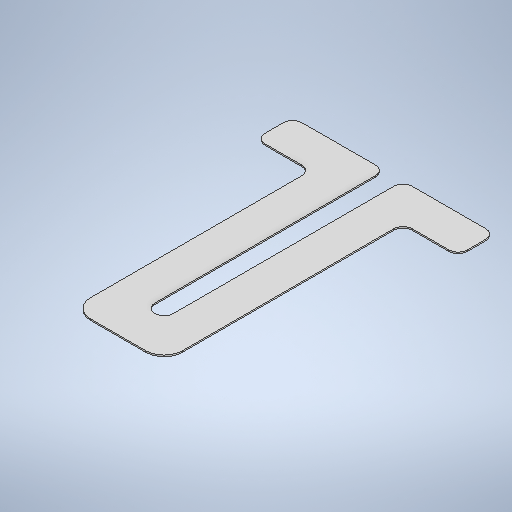
# Autodesk Inventor part: Part1
Saved by Autodesk Inventor 2025.4 (Build 294407000, 407)
## iProperties
Created: 2026-04-15
Part Number: Part1
Material: Generic
Document SubType Name: Modeling
Designer: gdira
Density: 1 g/cm^3
Appearance: Default
Author: gdira
Autodesk Inventor part; units mm, degrees
ref_plane "YZ Plane" through (0, 0, 0) normal (1, 0, 0) x (0, 1, 0)
ref_plane "XZ Plane" through (0, 0, 0) normal (0, 1, 0) x (-1, 0, 0)
ref_plane "XY Plane" through (0, 0, 0) normal (0, 0, 1) x (1, 0, 0)
sketch "Sketch1" plane through (0, 0, 0) normal (0, 1, 0) x (-1, 0, 0)
  line L0 (-7.6804, 9.5695) -> (-1.6804, 9.5695)
  line L1 (-4.6804, 5.5695) -> (-4.6804, 5.5695)
  line L2 (-0.6897, -20.436) -> (5.3214, -20.425)
  line L3 (-0.6897, -20.436) -> (-2.6804, -20.436)
  line L4 (-3.6804, -19.436) -> (-3.6804, 4.5695)
  line L5 (-5.6804, 4.5695) -> (-5.6804, -19.4328)
  line L6 (0.3196, 7.5695) -> (0.3196, -12.405)
  line L7 (-6.6804, -20.4328) -> (-14.6804, -20.4328)
  line L8 (-9.6804, 7.5695) -> (-9.6804, -12.4328)
  arc A0 (-7.6804, 9.5695) -> (-9.6804, 7.5695) centre (-7.6804, 7.5695) ccw
  arc A1 (0.3196, 7.5695) -> (-1.6804, 9.5695) centre (-1.6804, 7.5695) ccw
  line L9 (6.3196, -19.425) -> (6.3196, -17.4232)
  line L10 (5.3196, -16.4232) -> (1.3196, -16.4232)
  line L11 (0.3196, -15.4232) -> (0.3196, -8.8508)
  line L12 (-15.6804, -19.4328) -> (-15.6804, -17.4328)
  line L13 (-14.6804, -16.4328) -> (-10.6804, -16.4328)
  line L14 (-9.6804, -15.4328) -> (-9.6804, -12.4328)
  arc A2 (-10.6804, -16.4328) -> (-9.6804, -15.4328) centre (-10.6804, -15.4328) ccw
  arc A3 (-14.6804, -16.4328) -> (-15.6804, -17.4328) centre (-14.6804, -17.4328) ccw
  arc A4 (-15.6804, -19.4328) -> (-14.6804, -20.4328) centre (-14.6804, -19.4328) ccw
  arc A5 (-6.6804, -20.4328) -> (-5.6804, -19.4328) centre (-6.6804, -19.4328) ccw
  arc A6 (-3.6804, -19.436) -> (-2.6804, -20.436) centre (-2.6804, -19.436) ccw
  arc A7 (5.3214, -20.425) -> (6.3196, -19.425) centre (5.3196, -19.425) ccw
  arc A8 (6.3196, -17.4232) -> (5.3196, -16.4232) centre (5.3196, -17.4232) ccw
  arc A9 (0.3196, -15.4232) -> (1.3196, -16.4232) centre (1.3196, -15.4232) ccw
  arc A10 (-4.6804, 5.5695) -> (-5.6804, 4.5695) centre (-4.6804, 4.5695) ccw
  arc A11 (-3.6804, 4.5695) -> (-4.6804, 5.5695) centre (-4.6804, 4.5695) ccw
  point P0 (0, 0)
  point P1 (6.3196, -20.4232)
  point P2 (-3.6804, -20.436)
  point P3 (-15.6804, -20.4328)
  point P4 (-4.6804, 9.5695)
  point P5 (-4.6804, 5.5695)
  point P6 (2.3159, -20.4305)
  point P7 (6.3196, -16.4232)
  point P8 (-15.6804, -16.4328)
  point P9 (0.3196, -12.405)
  dimension "d0" = 10
  dimension "d2" = 4
  dimension "d3" = 4
  dimension "d4" = 2
  dimension "d5" = 4
  dimension "d6" = 30
  dimension "d7" = 2
  dimension "d8" = 4
  dimension "d9" = 4
  dimension "d10" = 1
  dimension "d11" = 1
  constraints: 30 end point, 24 point on circle, 24 tangent, 12 centre point, 11 point on line, 9 equal radius, 5 perpendicular, 3 midpoint, 2 horizontal, 2 vertical, 1 collinear, 1 parallel
  measures "d0" distance of point (6.32, -20.423) point (-3.68, -20.436)
  measures "d2" distance between parallel lines of L4 L6
  measures "d3" distance between parallel lines of L8 L5
  measures "d4" distance between parallel lines of L5 L4
  measures "d5" distance of point (-4.68, 9.57) point (-4.68, 5.57)
  measures "d6" distance from line of point (2.316, -20.43) L0
  measures "d7" radius of A0
  measures "d8" distance of point (6.32, -20.423) point (6.32, -16.423)
  measures "d9" distance of point (-15.68, -20.433) point (-15.68, -16.433)
  measures "d10" radius of A2
  measures "d11" radius of A10
extrude "Extrusion1" add sketch "Sketch1" along normal blind 0.15
body "Solid1"
